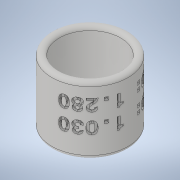
# Autodesk Inventor part: LargeFinderEyePieceCover
Saved by Autodesk Inventor 2021.1 (Build 251245000, 245)
## iProperties
Created: 2018-09-01
Part Number: LargeFinderEyePieceCover
Material: Generic
Document SubType Name: Modeling
Designer: steele
Density: 1 g/cm^3
Appearance: Default
Author: steele
Autodesk Inventor part; units mm, degrees
ref_plane "XZ Plane" through (0, 0, 0) normal (0, 1, 0) x (-1, 0, 0)
ref_plane "XY Plane" through (0, 0, 0) normal (0, 0, 1) x (1, 0, 0)
sketch "Sketch1" plane through (0, 0, 0) normal (0, 1, 0) x (-1, 0, 0)
  circle A0 centre (0, 0) radius 16.256
  dimension "d0" = 32.512
  constraints: 1 centre point, 1 coincident
  measures "d0" diameter of A0
extrude "Extrusion1" add sketch "Sketch1" along normal blind 3.175
sketch "Sketch2" plane through (0, 3.175, 0) normal (0, 1, 0) x (1, 0, 0)
  circle A0 centre (0, 0) radius 16.256
  circle A1 centre (0, 0) radius 13.081
  dimension "d3" = 32.512
  dimension "d4" = 26.162
  constraints: 2 centre point, 2 coincident
  measures "d3" diameter of A0
  measures "d4" diameter of A1
extrude "Extrusion2" add sketch "Sketch2" along normal blind 25.4
ref_plane "Work Plane1" through (16.256, 0, 0) normal (1, 0, 0) x (0, 1, 0)
sketch "Sketch3" plane through (16.256, 0, 0) normal (1, 0, 0) x (0, 1, 0)
  line L0 (0, 16.256) -> (28.575, 16.256) construction
  line L1 (14.2875, 16.256) -> (14.2875, -16.5017) construction
  line L2 (3.175, -13.081) -> (28.575, -13.081) construction
  line L3 (10.082, -14.834) -> (10.082, -15.7643)
  line L4 (10.082, -15.7643) -> (9.2075, -15.7643)
  line L5 (9.2075, -15.7643) -> (9.2075, -12.8363)
  line L6 (9.2075, -12.8363) -> (10.082, -12.8363)
  line L7 (10.082, -12.8363) -> (10.082, -13.7666)
  line L8 (10.082, -13.7666) -> (13.4087, -13.7666)
  line L9 (13.4087, -13.7666) -> (13.4087, -12.8363)
  line L10 (13.4087, -12.8363) -> (14.2875, -12.8363)
  line L11 (14.2875, -12.8363) -> (14.2875, -15.7643)
  line L12 (14.2875, -15.7643) -> (13.4087, -15.7643)
  line L13 (13.4087, -15.7643) -> (13.4087, -14.834)
  line L14 (13.4087, -14.834) -> (10.082, -14.834)
  spline S0 degree 2 poles (9.2075, -9.8912) (9.2075, -8.9653) (10.5021, -8.0007) (11.7454, -8.0007) knots 0 0 0 1 2 2 2
  spline S1 degree 2 poles (11.7454, -8.0007) (13.0057, -8.0007) (14.2875, -8.9567) (14.2875, -9.8912) knots 0 0 0 1 2 2 2
  line L15 (14.2875, -9.8912) -> (14.2875, -11.5846)
  line L16 (14.2875, -11.5846) -> (9.2075, -11.5846)
  line L17 (9.2075, -11.5846) -> (9.2075, -9.8912)
  line L18 (10.1506, -9.8912) -> (10.1506, -10.5085)
  line L19 (10.1506, -10.5085) -> (13.3358, -10.5085)
  line L20 (13.3358, -10.5085) -> (13.3358, -9.8912)
  spline S2 degree 2 poles (13.3358, -9.8912) (13.3358, -9.4754) (12.5942, -9.0981) (11.7454, -9.0981) knots 0 0 0 1 2 2 2
  spline S3 degree 2 poles (11.7454, -9.0981) (10.9566, -9.0981) (10.1506, -9.5011) (10.1506, -9.8912) knots 0 0 0 1 2 2 2
  line L21 (12.9414, -6.1487) -> (12.9414, -4.8027)
  line L22 (12.9414, -4.8027) -> (14.2875, -4.8027)
  line L23 (14.2875, -4.8027) -> (14.2875, -6.1487)
  line L24 (14.2875, -6.1487) -> (12.9414, -6.1487)
  line L25 (10.3564, -6.1487) -> (10.3564, -4.8027)
  line L26 (10.3564, -4.8027) -> (11.7025, -4.8027)
  line L27 (11.7025, -4.8027) -> (11.7025, -6.1487)
  line L28 (11.7025, -6.1487) -> (10.3564, -6.1487)
  line L29 (10.7894, 3.141) -> (10.7894, 1.9192)
  line L30 (10.7894, 1.9192) -> (10.0692, 1.9192)
  line L31 (10.0692, 1.9192) -> (10.0692, 1.9707)
  spline S4 degree 2 poles (10.0692, 1.9707) (10.0692, 2.6737) (9.6705, 3.2696) (9.1689, 3.3296) knots 0 0 0 1 2 2 2
  line L32 (9.1689, 3.3296) -> (9.1689, 4.1527)
  line L33 (9.1689, 4.1527) -> (14.2875, 4.1527)
  line L34 (14.2875, 4.1527) -> (14.2875, 3.141)
  line L35 (14.2875, 3.141) -> (10.7894, 3.141)
  line L36 (12.9414, 7.085) -> (12.9414, 8.4311)
  line L37 (12.9414, 8.4311) -> (14.2875, 8.4311)
  line L38 (14.2875, 8.4311) -> (14.2875, 7.085)
  line L39 (14.2875, 7.085) -> (12.9414, 7.085)
  spline S5 degree 2 poles (11.7325, 10.3173) (10.4721, 10.3173) (9.1689, 11.2561) (9.1689, 12.1693) knots 0 0 0 1 2 2 2
  spline S6 degree 2 poles (9.1689, 12.1693) (9.1689, 13.0952) (10.485, 14.0169) (11.8097, 14.0169) knots 0 0 0 1 2 2 2
  spline S7 degree 2 poles (11.8097, 14.0169) (13.13, 14.0169) (14.429, 13.1038) (14.429, 12.1693) knots 0 0 0 1 2 2 2
  spline S8 degree 2 poles (14.429, 12.1693) (14.429, 11.2304) (13.1043, 10.3173) (11.7325, 10.3173) knots 0 0 0 1 2 2 2
  spline S9 degree 2 poles (10.0263, 12.1607) (10.0263, 11.762) (10.8623, 11.3805) (11.7368, 11.3805) knots 0 0 0 1 2 2 2
  spline S10 degree 2 poles (11.7368, 11.3805) (12.7185, 11.3805) (13.5759, 11.7491) (13.5759, 12.1607) knots 0 0 0 1 2 2 2
  spline S11 degree 2 poles (13.5759, 12.1607) (13.5759, 12.5722) (12.7271, 12.9538) (11.8011, 12.9538) knots 0 0 0 1 2 2 2
  spline S12 degree 2 poles (11.8011, 12.9538) (10.8708, 12.9538) (10.0263, 12.5722) (10.0263, 12.1607) knots 0 0 0 1 2 2 2
  spline S13 degree 2 poles (12.7271, 15.6974) (13.1429, 15.6974) (13.5887, 16.0961) (13.5887, 16.4733) knots 0 0 0 1 2 2 2
  spline S14 degree 2 poles (13.5887, 16.4733) (13.5887, 16.8849) (13.19, 17.305) (12.8042, 17.305) knots 0 0 0 1 2 2 2
  spline S15 degree 2 poles (12.8042, 17.305) (12.4184, 17.305) (12.0454, 16.8163) (12.0454, 16.2976) knots 0 0 0 1 2 2 2
  line L40 (12.0454, 16.2976) -> (12.0454, 16.1775)
  line L41 (12.0454, 16.1775) -> (11.3381, 16.1775)
  line L42 (11.3381, 16.1775) -> (11.3381, 16.289)
  spline S16 degree 2 poles (11.3381, 16.289) (11.3381, 16.7305) (10.9909, 17.1635) (10.6308, 17.1635) knots 0 0 0 1 2 2 2
  spline S17 degree 2 poles (10.6308, 17.1635) (10.335, 17.1635) (9.9877, 16.7949) (9.9877, 16.4862) knots 0 0 0 1 2 2 2
  spline S18 degree 2 poles (9.9877, 16.4862) (9.9877, 16.1475) (10.3821, 15.7831) (10.7551, 15.7831) knots 0 0 0 1 2 2 2
  line L43 (10.7551, 15.7831) -> (10.7979, 15.7831)
  line L44 (10.7979, 15.7831) -> (10.7979, 14.8186)
  spline S19 degree 2 poles (10.7979, 14.8186) (10.0177, 14.8272) (9.1732, 15.7188) (9.1732, 16.5291) knots 0 0 0 1 2 2 2
  spline S20 degree 2 poles (9.1732, 16.5291) (9.1732, 17.2964) (9.9234, 18.2052) (10.5622, 18.2052) knots 0 0 0 1 2 2 2
  spline S21 degree 2 poles (10.5622, 18.2052) (10.8965, 18.2052) (11.4067, 17.8966) (11.5696, 17.5922) knots 0 0 0 1 2 2 2
  spline S22 degree 2 poles (11.5696, 17.5922) (11.7411, 17.9823) (12.3455, 18.381) (12.7656, 18.381) knots 0 0 0 1 2 2 2
  spline S23 degree 2 poles (12.7656, 18.381) (13.533, 18.381) (14.4333, 17.365) (14.4333, 16.5033) knots 0 0 0 1 2 2 2
  spline S24 degree 2 poles (14.4333, 16.5033) (14.4333, 15.6417) (13.5544, 14.7071) (12.7399, 14.7071) knots 0 0 0 1 2 2 2
  line L45 (12.7399, 14.7071) -> (12.7271, 14.7071)
  line L46 (12.7271, 14.7071) -> (12.7271, 15.6974)
  spline S25 degree 2 poles (11.7325, 19.1398) (10.4721, 19.1398) (9.1689, 20.0786) (9.1689, 20.9917) knots 0 0 0 1 2 2 2
  spline S26 degree 2 poles (9.1689, 20.9917) (9.1689, 21.9177) (10.485, 22.8394) (11.8097, 22.8394) knots 0 0 0 1 2 2 2
  spline S27 degree 2 poles (11.8097, 22.8394) (13.13, 22.8394) (14.429, 21.9263) (14.429, 20.9917) knots 0 0 0 1 2 2 2
  spline S28 degree 2 poles (14.429, 20.9917) (14.429, 20.0529) (13.1043, 19.1398) (11.7325, 19.1398) knots 0 0 0 1 2 2 2
  spline S29 degree 2 poles (10.0263, 20.9832) (10.0263, 20.5845) (10.8623, 20.203) (11.7368, 20.203) knots 0 0 0 1 2 2 2
  spline S30 degree 2 poles (11.7368, 20.203) (12.7185, 20.203) (13.5759, 20.5716) (13.5759, 20.9832) knots 0 0 0 1 2 2 2
  spline S31 degree 2 poles (13.5759, 20.9832) (13.5759, 21.3947) (12.7271, 21.7763) (11.8011, 21.7763) knots 0 0 0 1 2 2 2
  spline S32 degree 2 poles (11.8011, 21.7763) (10.8708, 21.7763) (10.0263, 21.3947) (10.0263, 20.9832) knots 0 0 0 1 2 2 2
  spline S33 degree 2 poles (20.1171, -16.1801) (18.8997, -16.1801) (17.4893, -15.1641) (17.4893, -14.2982) knots 0 0 0 1 2 2 2
  spline S34 degree 2 poles (17.4893, -14.2982) (17.4893, -13.4194) (18.9168, -12.4162) (20.1686, -12.4162) knots 0 0 0 1 2 2 2
  spline S35 degree 2 poles (20.1686, -12.4162) (21.4247, -12.4162) (22.8522, -13.4194) (22.8522, -14.2982) knots 0 0 0 1 2 2 2
  spline S36 degree 2 poles (22.8522, -14.2982) (22.8522, -15.1856) (21.4161, -16.1801) (20.1171, -16.1801) knots 0 0 0 1 2 2 2
  spline S37 degree 2 poles (18.4324, -14.3025) (18.4324, -14.6754) (19.2726, -15.0913) (20.0443, -15.0913) knots 0 0 0 1 2 2 2
  spline S38 degree 2 poles (20.0443, -15.0913) (21.0003, -15.0913) (21.8919, -14.7012) (21.8919, -14.281) knots 0 0 0 1 2 2 2
  spline S39 degree 2 poles (21.8919, -14.281) (21.8919, -13.8909) (21.0646, -13.5137) (20.1814, -13.5137) knots 0 0 0 1 2 2 2
  spline S40 degree 2 poles (20.1814, -13.5137) (19.2983, -13.5137) (18.4324, -13.9038) (18.4324, -14.3025) knots 0 0 0 1 2 2 2
  spline S41 degree 2 poles (17.6307, -9.8912) (17.6307, -8.9653) (18.9254, -8.0007) (20.1686, -8.0007) knots 0 0 0 1 2 2 2
  spline S42 degree 2 poles (20.1686, -8.0007) (21.4289, -8.0007) (22.7107, -8.9567) (22.7107, -9.8912) knots 0 0 0 1 2 2 2
  line L47 (22.7107, -9.8912) -> (22.7107, -11.5846)
  line L48 (22.7107, -11.5846) -> (17.6307, -11.5846)
  line L49 (17.6307, -11.5846) -> (17.6307, -9.8912)
  line L50 (18.5739, -9.8912) -> (18.5739, -10.5085)
  line L51 (18.5739, -10.5085) -> (21.759, -10.5085)
  line L52 (21.759, -10.5085) -> (21.759, -9.8912)
  spline S43 degree 2 poles (21.759, -9.8912) (21.759, -9.4754) (21.0174, -9.0981) (20.1686, -9.0981) knots 0 0 0 1 2 2 2
  spline S44 degree 2 poles (20.1686, -9.0981) (19.3798, -9.0981) (18.5739, -9.5011) (18.5739, -9.8912) knots 0 0 0 1 2 2 2
  line L53 (18.7796, -6.1487) -> (18.7796, -4.8027)
  line L54 (18.7796, -4.8027) -> (20.1257, -4.8027)
  line L55 (20.1257, -4.8027) -> (20.1257, -6.1487)
  line L56 (20.1257, -6.1487) -> (18.7796, -6.1487)
  line L57 (21.3646, -6.1487) -> (21.3646, -4.8027)
  line L58 (21.3646, -4.8027) -> (22.7107, -4.8027)
  line L59 (22.7107, -4.8027) -> (22.7107, -6.1487)
  line L60 (22.7107, -6.1487) -> (21.3646, -6.1487)
  line L61 (19.2126, 3.141) -> (19.2126, 1.9192)
  line L62 (19.2126, 1.9192) -> (18.4924, 1.9192)
  line L63 (18.4924, 1.9192) -> (18.4924, 1.9707)
  spline S45 degree 2 poles (18.4924, 1.9707) (18.4924, 2.6737) (18.0937, 3.2696) (17.5921, 3.3296) knots 0 0 0 1 2 2 2
  line L64 (17.5921, 3.3296) -> (17.5921, 4.1527)
  line L65 (17.5921, 4.1527) -> (22.7107, 4.1527)
  line L66 (22.7107, 4.1527) -> (22.7107, 3.141)
  line L67 (22.7107, 3.141) -> (19.2126, 3.141)
  line L68 (21.3646, 7.085) -> (21.3646, 8.4311)
  line L69 (21.3646, 8.4311) -> (22.7107, 8.4311)
  line L70 (22.7107, 8.4311) -> (22.7107, 7.085)
  line L71 (22.7107, 7.085) -> (21.3646, 7.085)
  line L72 (19.4227, 11.3333) -> (19.4227, 10.3902)
  line L73 (19.4227, 10.3902) -> (19.4012, 10.3902)
  spline S46 degree 2 poles (19.4012, 10.3902) (18.5567, 10.3902) (17.5921, 11.329) (17.5921, 12.1521) knots 0 0 0 1 2 2 2
  spline S47 degree 2 poles (17.5921, 12.1521) (17.5921, 12.9838) (18.4452, 13.9483) (19.1654, 13.9483) knots 0 0 0 1 2 2 2
  spline S48 degree 2 poles (19.1654, 13.9483) (19.6799, 13.9483) (20.4472, 13.4425) (20.9059, 12.7394) knots 0 0 0 1 2 2 2
  spline S49 degree 2 poles (20.9059, 12.7394) (21.0045, 12.598) (21.1632, 12.345) knots 0 0 0 1 1 1
  spline S50 degree 2 poles (21.1632, 12.345) (21.6047, 11.6505) (21.8362, 11.5691) knots 0 0 0 1 1 1
  line L74 (21.8362, 11.5691) -> (21.8362, 13.8969)
  line L75 (21.8362, 13.8969) -> (22.7107, 13.8969)
  line L76 (22.7107, 13.8969) -> (22.7107, 10.3045)
  spline S51 degree 2 poles (22.7107, 10.3045) (22.012, 10.3173) (21.0731, 10.8832) (20.5801, 11.6163) knots 0 0 0 1 2 2 2
  spline S52 degree 2 poles (20.5801, 11.6163) (20.503, 11.7277) (20.3658, 11.9421) knots 0 0 0 1 1 1
  spline S53 degree 2 poles (20.3658, 11.9421) (19.757, 12.9023) (19.1826, 12.9023) knots 0 0 0 1 1 1
  spline S54 degree 2 poles (19.1826, 12.9023) (18.8482, 12.9023) (18.4495, 12.4908) (18.4495, 12.1393) knots 0 0 0 1 2 2 2
  spline S55 degree 2 poles (18.4495, 12.1393) (18.4495, 11.7577) (18.934, 11.3333) (19.3798, 11.3333) knots 0 0 0 1 2 2 2
  line L77 (19.3798, 11.3333) -> (19.4227, 11.3333)
  spline S56 degree 2 poles (20.0185, 17.6737) (20.2029, 18.0466) (20.8159, 18.4153) (21.2575, 18.4153) knots 0 0 0 1 2 2 2
  spline S57 degree 2 poles (21.2575, 18.4153) (22.0077, 18.4153) (22.8565, 17.4379) (22.8565, 16.5805) knots 0 0 0 1 2 2 2
  spline S58 degree 2 poles (22.8565, 16.5805) (22.8565, 15.7103) (22.012, 14.7414) (21.2575, 14.7414) knots 0 0 0 1 2 2 2
  spline S59 degree 2 poles (21.2575, 14.7414) (20.8116, 14.7414) (20.2243, 15.1015) (20.0185, 15.4916) knots 0 0 0 1 2 2 2
  spline S60 degree 2 poles (20.0185, 15.4916) (19.8428, 15.1701) (19.3712, 14.8829) (19.0111, 14.8829) knots 0 0 0 1 2 2 2
  spline S61 degree 2 poles (19.0111, 14.8829) (18.3424, 14.8829) (17.5836, 15.7831) (17.5836, 16.5805) knots 0 0 0 1 2 2 2
  spline S62 degree 2 poles (17.5836, 16.5805) (17.5836, 17.3779) (18.3295, 18.2781) (18.9897, 18.2781) knots 0 0 0 1 2 2 2
  spline S63 degree 2 poles (18.9897, 18.2781) (19.3541, 18.2781) (19.8642, 17.978) (20.0185, 17.6737) knots 0 0 0 1 2 2 2
  spline S64 degree 2 poles (20.4387, 16.5805) (20.4387, 16.2204) (20.8845, 15.7831) (21.2575, 15.7831) knots 0 0 0 1 2 2 2
  spline S65 degree 2 poles (21.2575, 15.7831) (21.6133, 15.7831) (22.0077, 16.2033) (22.0077, 16.5805) knots 0 0 0 1 2 2 2
  spline S66 degree 2 poles (22.0077, 16.5805) (22.0077, 16.9578) (21.5918, 17.3864) (21.2232, 17.3864) knots 0 0 0 1 2 2 2
  spline S67 degree 2 poles (21.2232, 17.3864) (20.8759, 17.3864) (20.4387, 16.9406) (20.4387, 16.5805) knots 0 0 0 1 2 2 2
  spline S68 degree 2 poles (18.411, 16.5805) (18.411, 16.2504) (18.7453, 15.8603) (19.024, 15.8603) knots 0 0 0 1 2 2 2
  spline S69 degree 2 poles (19.024, 15.8603) (19.3198, 15.8603) (19.6413, 16.2333) (19.6413, 16.5805) knots 0 0 0 1 2 2 2
  spline S70 degree 2 poles (19.6413, 16.5805) (19.6413, 16.9277) (19.3198, 17.3007) (19.024, 17.3007) knots 0 0 0 1 2 2 2
  spline S71 degree 2 poles (19.024, 17.3007) (18.7453, 17.3007) (18.411, 16.9149) (18.411, 16.5805) knots 0 0 0 1 2 2 2
  spline S72 degree 2 poles (20.1557, 19.1398) (18.8954, 19.1398) (17.5921, 20.0786) (17.5921, 20.9917) knots 0 0 0 1 2 2 2
  spline S73 degree 2 poles (17.5921, 20.9917) (17.5921, 21.9177) (18.9082, 22.8394) (20.2329, 22.8394) knots 0 0 0 1 2 2 2
  spline S74 degree 2 poles (20.2329, 22.8394) (21.5533, 22.8394) (22.8522, 21.9263) (22.8522, 20.9917) knots 0 0 0 1 2 2 2
  spline S75 degree 2 poles (22.8522, 20.9917) (22.8522, 20.0529) (21.5275, 19.1398) (20.1557, 19.1398) knots 0 0 0 1 2 2 2
  spline S76 degree 2 poles (18.4495, 20.9832) (18.4495, 20.5845) (19.2855, 20.203) (20.16, 20.203) knots 0 0 0 1 2 2 2
  spline S77 degree 2 poles (20.16, 20.203) (21.1417, 20.203) (21.9991, 20.5716) (21.9991, 20.9832) knots 0 0 0 1 2 2 2
  spline S78 degree 2 poles (21.9991, 20.9832) (21.9991, 21.3947) (21.1503, 21.7763) (20.2243, 21.7763) knots 0 0 0 1 2 2 2
  spline S79 degree 2 poles (20.2243, 21.7763) (19.2941, 21.7763) (18.4495, 21.3947) (18.4495, 20.9832) knots 0 0 0 1 2 2 2
  point P0 (0, 0)
  constraints: 2 end point, 1 midpoint, 1 perpendicular, 1 vertical
emboss "Emboss1" sketch "Sketch3" operation cut depth 1.27 direction (1, 0, 0) wrap yes faces at (-16.0455, 10.5833, -2.6076)
fillet "Fillet1" radius 1.5875 1 edges at (16.256, 0, 0)
fillet "Fillet2" radius 1.5875 2 edges at (-13.081, 28.575, 0) (-16.256, 28.575, 0)
equation "\"d0\" = coverOD"
equation "\"d1\" = wallThickness"
equation "\"d3\" = coverOD"
equation "\"d4\" = eypPieceCoverID"
equation "\"d7\" = textDepth"
equation "\"d9\" = filletRadius"
equation "\"d10\" = filletRadius"
equation "\"wallThickness\" = 3.175"
equation "\"coverOD\" = eypPieceCoverID + 2 * wallThickness"
equation "\"eypPieceCoverID\" = 26.162"
equation "\"textDepth\" = 1.27"
equation "\"filletRadius\" = 1.5875"
body "Solid1"
